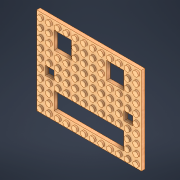
# Autodesk Inventor part: 0401_練習1
Saved by Autodesk Inventor 2022 (Build 260153000, 153)
## iProperties
Created: 2022-04-01
Part Number: 0401_練習1
Material: 一般
Document SubType Name: Modeling
Designer: User
Density: 1 g/cm^3
Appearance: 櫻桃木 - 天然低亮度
Author: User
Autodesk Inventor part; units mm, degrees
ref_plane "YZ Plane" through (0, 0, 0) normal (1, 0, 0) x (0, 1, 0)
ref_plane "XZ Plane" through (0, 0, 0) normal (0, 1, 0) x (-1, 0, 0)
ref_plane "XY Plane" through (0, 0, 0) normal (0, 0, 1) x (1, 0, 0)
sketch "草圖1" plane through (0, 0, 0) normal (0, 1, 0) x (-1, 0, 0)
  line L0 (0, 0) -> (-80, 0)
  line L1 (-80, 0) -> (-80, -96)
  line L2 (-80, -96) -> (0, -96)
  line L3 (0, -96) -> (0, 0)
  dimension "長" = 80
  dimension "寬" = 96
  constraints: 8 end point, 2 parallel, 1 horizontal, 1 perpendicular
  measures "長" distance of L2.end L1.end
  measures "寬" distance of L1.end L0.end
extrude "樂高擠出" add sketch "草圖1" against normal blind 3.2
sketch "草圖2" plane through (0, 0, 0) normal (0, 1, 0) x (-1, 0, 0)
  circle A0 centre (-76, -4) radius 2.5
  line L0 (-80, 0) -> (-80, -96) projected
  line L1 (0, 0) -> (-80, 0) projected
  dimension "d4" = 5
  dimension "d5" = 4
  dimension "d6" = 4
  constraints: 1 centre point
  measures "d4" diameter of A0
  measures "d5" distance from line of L0 A0.centre
  measures "d6" distance from line of L1 A0.centre
extrude "圓柱擠出" add sketch "草圖2" along normal blind 1.5
pattern_linear "頂部圓柱" count 12 spacing 8 along (0, 0, -1) count 10 spacing 8 along (-1, 0, 0) of "圓柱擠出"
shell "背面薄殼" thickness 1 removed faces 1 at (53.3333, -3.2, -32)
sketch "草圖3" plane through (1, -1, -1) normal (0, -1, 0) x (1, 0, 0)
  circle A0 centre (75, -3) radius 2.5 projected
  circle A1 centre (67, -3) radius 2.5 projected
  circle A2 centre (67, -11) radius 2.5 projected
  circle A3 centre (71, -7) radius 3.1569
  line L0 (78, -94) -> (0, -94) projected
  line L1 (78, -94) -> (0, -94) projected
  line L2 (78, 0) -> (78, -94) projected
  circle A4 centre (67, -19) radius 1.5 projected
  circle A5 centre (67, -11) radius 1.5 projected
  circle A6 centre (67, -3) radius 1.5 projected
  circle A7 centre (75, -19) radius 1.5 projected
  circle A8 centre (75, -11) radius 1.5 projected
  circle A9 centre (75, -3) radius 1.5 projected
  line L3 (78, 0) -> (78, -94) projected
  line L4 (0, 0) -> (78, 0) projected
  line L5 (0, -94) -> (0, 0) projected
  line L6 (78, -94) -> (0, -94) projected
  circle A10 centre (71, -15) radius 3.1569
  circle A11 centre (71, -7) radius 2.1569
  circle A12 centre (71, -15) radius 2.1569
  point P0 (-1, 1)
  dimension "d18" = 8
  dimension "d23" = 1
  dimension "d25" = 1
  constraints: 4 centre point, 3 tangent, 1 vertical, 2 other
  measures "d18" distance of A3.centre A10.centre
  measures "d23" radial gap between concentric circles of A3 A11
  measures "d25" radial gap between concentric circles of A10 A12
extrude "背面圓柱擠出" add sketch "草圖3" along normal up to surface (2.2 mm away) contours A3
pattern_linear "背面圓柱" count 11 spacing 8 along (0, 0, -1) count 9 spacing 8 along (-1, 0, 0) of "背面圓柱擠出"
sketch "草圖4" plane through (0, 0, 0) normal (0, 1, 0) x (1, 0, 0)
  circle A0 centre (8, 16) radius 2.1569 projected
  circle A1 centre (24, 32) radius 2.1569 projected
  line L0 (8, 16) -> (24, 16)
  line L1 (24, 16) -> (24, 32)
  line L2 (24, 32) -> (8, 32)
  line L3 (8, 32) -> (8, 16)
  circle A2 centre (24, 80) radius 2.1569 projected
  circle A3 centre (8, 64) radius 2.1569 projected
  line L4 (24, 80) -> (8, 80)
  line L5 (8, 80) -> (8, 64)
  line L6 (8, 64) -> (24, 64)
  line L7 (24, 64) -> (24, 80)
  circle A4 centre (72, 80) radius 2.1569 projected
  circle A5 centre (56, 16) radius 2.1569 projected
  line L8 (72, 80) -> (56, 80)
  line L9 (56, 80) -> (56, 16)
  line L10 (56, 16) -> (72, 16)
  line L11 (72, 16) -> (72, 80)
  circle A6 centre (40, 8) radius 2.1569 projected
  circle A7 centre (48, 16) radius 2.1569 projected
  line L12 (40, 8) -> (48, 8)
  line L13 (48, 8) -> (48, 16)
  line L14 (48, 16) -> (40, 16)
  line L15 (40, 16) -> (40, 8)
  circle A8 centre (40, 80) radius 2.1569 projected
  circle A9 centre (48, 88) radius 3.1569 projected
  line L16 (40, 80) -> (48, 80)
  line L17 (48, 80) -> (48, 88)
  line L18 (48, 88) -> (40, 88)
  line L19 (40, 88) -> (40, 80)
  point P0 (0, 0)
  point P1 (40, 10.1569)
  point P2 (42.1569, 8)
  point P3 (48, 13.8431)
  point P4 (45.8431, 16)
  point P5 (72, 77.8431)
  point P6 (69.8431, 80)
  point P7 (56, 18.1569)
  point P8 (58.1569, 16)
  point P9 (24, 77.8431)
  point P10 (21.8431, 80)
  point P11 (8, 66.1569)
  point P12 (10.1569, 64)
  point P13 (8, 18.1569)
  point P14 (10.1569, 16)
  point P15 (24, 29.8431)
  point P16 (21.8431, 32)
  constraints: 40 end point, 10 parallel, 5 horizontal, 5 perpendicular
extrude "表情切割" cut sketch "草圖4" along normal through all both and the other way through all contours A0 L3 L2 A1 L1 L0 | A2 L7 L6 A3 L5 L4 | A4 L11 L10 A5 L9 L8 | A6 L15 L14 A7 L13 L12 | L16 L19 A8 | A8 L19 L18 A9 L17 L16 | A9 L18 L17 picked at (40.4719, 81.3487) picked at (45.9218, 87.7658)
sketch "草圖5" plane through (1, -1, -1) normal (0, -1, 0) x (1, 0, 0)
  line L0 (47, -82.1569) -> (47, -83.8431) projected
  arc A0 (43.8431, -87) -> (47, -83.8431) centre (47, -87) ccw projected
  line L1 (43.8431, -87) -> (42.1569, -87) projected
  arc A1 (39, -83.8431) -> (42.1569, -87) centre (39, -87) ccw projected
  line L2 (39, -83.8431) -> (39, -82.1569) projected
  arc A2 (42.1569, -79) -> (39, -82.1569) centre (39, -79) ccw projected
  line L3 (42.1569, -79) -> (43.8431, -79) projected
  arc A3 (47, -82.1569) -> (43.8431, -79) centre (47, -79) ccw projected
  line L4 (43.8431, -15) -> (42.1569, -15) projected
  arc A4 (39, -11.8431) -> (42.1569, -15) centre (39, -15) ccw projected
  line L5 (39, -11.8431) -> (39, -10.1569) projected
  arc A5 (42.1569, -7) -> (39, -10.1569) centre (39, -7) ccw projected
  line L6 (42.1569, -7) -> (43.8431, -7) projected
  arc A6 (47, -10.1569) -> (43.8431, -7) centre (47, -7) ccw projected
  line L7 (47, -10.1569) -> (47, -11.8431) projected
  arc A7 (43.8431, -15) -> (47, -11.8431) centre (47, -15) ccw projected
  line L8 (11.8431, -31) -> (10.1569, -31) projected
  arc A8 (7, -27.8431) -> (10.1569, -31) centre (7, -31) ccw projected
  line L9 (7, -27.8431) -> (7, -26.1569) projected
  arc A9 (7, -19.8431) -> (7, -26.1569) centre (7, -23) ccw projected
  line L10 (7, -19.8431) -> (7, -18.1569) projected
  arc A10 (10.1569, -15) -> (7, -18.1569) centre (7, -15) ccw projected
  line L11 (10.1569, -15) -> (11.8431, -15) projected
  arc A11 (18.1569, -15) -> (11.8431, -15) centre (15, -15) ccw projected
  line L12 (18.1569, -15) -> (19.8431, -15) projected
  arc A12 (23, -18.1569) -> (19.8431, -15) centre (23, -15) ccw projected
  line L13 (23, -18.1569) -> (23, -19.8431) projected
  arc A13 (23, -26.1569) -> (23, -19.8431) centre (23, -23) ccw projected
  line L14 (23, -26.1569) -> (23, -27.8431) projected
  arc A14 (19.8431, -31) -> (23, -27.8431) centre (23, -31) ccw projected
  line L15 (19.8431, -31) -> (18.1569, -31) projected
  arc A15 (11.8431, -31) -> (18.1569, -31) centre (15, -31) ccw projected
  circle A16 centre (7, -87) radius 3.1569 projected
  circle A17 centre (7, -55) radius 3.1569 projected
  circle A18 centre (7, -47) radius 3.1569 projected
  circle A19 centre (7, -39) radius 3.1569 projected
  circle A20 centre (7, -7) radius 3.1569 projected
  circle A21 centre (15, -87) radius 3.1569 projected
  circle A22 centre (15, -55) radius 3.1569 projected
  circle A23 centre (15, -47) radius 3.1569 projected
  circle A24 centre (15, -39) radius 3.1569 projected
  circle A25 centre (15, -7) radius 3.1569 projected
  circle A26 centre (23, -87) radius 3.1569 projected
  line L16 (10.1569, -63) -> (11.8431, -63) projected
  arc A27 (18.1569, -63) -> (11.8431, -63) centre (15, -63) ccw projected
  line L17 (18.1569, -63) -> (19.8431, -63) projected
  arc A28 (23, -66.1569) -> (19.8431, -63) centre (23, -63) ccw projected
  line L18 (23, -66.1569) -> (23, -67.8431) projected
  arc A29 (23, -74.1569) -> (23, -67.8431) centre (23, -71) ccw projected
  line L19 (23, -74.1569) -> (23, -75.8431) projected
  arc A30 (19.8431, -79) -> (23, -75.8431) centre (23, -79) ccw projected
  line L20 (19.8431, -79) -> (18.1569, -79) projected
  arc A31 (11.8431, -79) -> (18.1569, -79) centre (15, -79) ccw projected
  line L21 (11.8431, -79) -> (10.1569, -79) projected
  arc A32 (7, -75.8431) -> (10.1569, -79) centre (7, -79) ccw projected
  line L22 (7, -75.8431) -> (7, -74.1569) projected
  arc A33 (7, -67.8431) -> (7, -74.1569) centre (7, -71) ccw projected
  line L23 (7, -67.8431) -> (7, -66.1569) projected
  arc A34 (10.1569, -63) -> (7, -66.1569) centre (7, -63) ccw projected
  circle A35 centre (23, -55) radius 3.1569 projected
  circle A36 centre (23, -47) radius 3.1569 projected
  circle A37 centre (23, -39) radius 3.1569 projected
  circle A38 centre (23, -7) radius 3.1569 projected
  circle A39 centre (31, -87) radius 3.1569 projected
  circle A40 centre (31, -79) radius 3.1569 projected
  circle A41 centre (31, -71) radius 3.1569 projected
  circle A42 centre (31, -63) radius 3.1569 projected
  circle A43 centre (31, -55) radius 3.1569 projected
  circle A44 centre (31, -47) radius 3.1569 projected
  circle A45 centre (31, -39) radius 3.1569 projected
  circle A46 centre (31, -31) radius 3.1569 projected
  circle A47 centre (31, -23) radius 3.1569 projected
  circle A48 centre (31, -15) radius 3.1569 projected
  circle A49 centre (31, -7) radius 3.1569 projected
  circle A50 centre (39, -71) radius 3.1569 projected
  circle A51 centre (39, -63) radius 3.1569 projected
  circle A52 centre (39, -55) radius 3.1569 projected
  circle A53 centre (39, -47) radius 3.1569 projected
  circle A54 centre (39, -39) radius 3.1569 projected
  circle A55 centre (39, -31) radius 3.1569 projected
  circle A56 centre (39, -23) radius 3.1569 projected
  circle A57 centre (47, -71) radius 3.1569 projected
  circle A58 centre (47, -63) radius 3.1569 projected
  circle A59 centre (47, -55) radius 3.1569 projected
  circle A60 centre (47, -47) radius 3.1569 projected
  circle A61 centre (47, -39) radius 3.1569 projected
  circle A62 centre (47, -31) radius 3.1569 projected
  circle A63 centre (47, -23) radius 3.1569 projected
  circle A64 centre (55, -87) radius 3.1569 projected
  circle A65 centre (55, -7) radius 3.1569 projected
  circle A66 centre (63, -87) radius 3.1569 projected
  circle A67 centre (63, -7) radius 3.1569 projected
  circle A68 centre (71, -87) radius 3.1569 projected
  line L24 (58.1569, -15) -> (59.8431, -15) projected
  arc A69 (66.1569, -15) -> (59.8431, -15) centre (63, -15) ccw projected
  line L25 (66.1569, -15) -> (67.8431, -15) projected
  arc A70 (71, -18.1569) -> (67.8431, -15) centre (71, -15) ccw projected
  line L26 (71, -18.1569) -> (71, -19.8431) projected
  arc A71 (71, -26.1569) -> (71, -19.8431) centre (71, -23) ccw projected
  line L27 (71, -26.1569) -> (71, -27.8431) projected
  arc A72 (71, -34.1569) -> (71, -27.8431) centre (71, -31) ccw projected
  line L28 (71, -34.1569) -> (71, -35.8431) projected
  arc A73 (71, -42.1569) -> (71, -35.8431) centre (71, -39) ccw projected
  line L29 (71, -42.1569) -> (71, -43.8431) projected
  arc A74 (71, -50.1569) -> (71, -43.8431) centre (71, -47) ccw projected
  line L30 (71, -50.1569) -> (71, -51.8431) projected
  arc A75 (71, -58.1569) -> (71, -51.8431) centre (71, -55) ccw projected
  line L31 (71, -58.1569) -> (71, -59.8431) projected
  arc A76 (71, -66.1569) -> (71, -59.8431) centre (71, -63) ccw projected
  line L32 (71, -66.1569) -> (71, -67.8431) projected
  arc A77 (71, -74.1569) -> (71, -67.8431) centre (71, -71) ccw projected
  line L33 (71, -74.1569) -> (71, -75.8431) projected
  arc A78 (67.8431, -79) -> (71, -75.8431) centre (71, -79) ccw projected
  line L34 (67.8431, -79) -> (66.1569, -79) projected
  arc A79 (59.8431, -79) -> (66.1569, -79) centre (63, -79) ccw projected
  line L35 (59.8431, -79) -> (58.1569, -79) projected
  arc A80 (55, -75.8431) -> (58.1569, -79) centre (55, -79) ccw projected
  line L36 (55, -75.8431) -> (55, -74.1569) projected
  arc A81 (55, -67.8431) -> (55, -74.1569) centre (55, -71) ccw projected
  line L37 (55, -67.8431) -> (55, -66.1569) projected
  arc A82 (55, -59.8431) -> (55, -66.1569) centre (55, -63) ccw projected
  line L38 (55, -59.8431) -> (55, -58.1569) projected
  arc A83 (55, -51.8431) -> (55, -58.1569) centre (55, -55) ccw projected
  line L39 (55, -51.8431) -> (55, -50.1569) projected
  arc A84 (55, -43.8431) -> (55, -50.1569) centre (55, -47) ccw projected
  line L40 (55, -43.8431) -> (55, -42.1569) projected
  arc A85 (55, -35.8431) -> (55, -42.1569) centre (55, -39) ccw projected
  line L41 (55, -35.8431) -> (55, -34.1569) projected
  arc A86 (55, -27.8431) -> (55, -34.1569) centre (55, -31) ccw projected
  line L42 (55, -27.8431) -> (55, -26.1569) projected
  arc A87 (55, -19.8431) -> (55, -26.1569) centre (55, -23) ccw projected
  line L43 (55, -19.8431) -> (55, -18.1569) projected
  arc A88 (58.1569, -15) -> (55, -18.1569) centre (55, -15) ccw projected
  line L44 (78, 0) -> (78, -94) projected
  line L45 (0, 0) -> (78, 0) projected
  line L46 (0, -94) -> (0, 0) projected
  line L47 (78, -94) -> (0, -94) projected
  circle A89 centre (75, -3) radius 1.5 projected
  circle A90 centre (75, -11) radius 1.5 projected
  circle A91 centre (75, -19) radius 1.5 projected
  circle A92 centre (75, -27) radius 1.5 projected
  circle A93 centre (75, -35) radius 1.5 projected
  circle A94 centre (75, -43) radius 1.5 projected
  circle A95 centre (75, -51) radius 1.5 projected
  circle A96 centre (75, -59) radius 1.5 projected
  circle A97 centre (75, -67) radius 1.5 projected
  circle A98 centre (75, -75) radius 1.5 projected
  circle A99 centre (75, -83) radius 1.5 projected
  circle A100 centre (75, -91) radius 1.5 projected
  circle A101 centre (67, -3) radius 1.5 projected
  circle A102 centre (67, -11) radius 1.5 projected
  circle A103 centre (67, -83) radius 1.5 projected
  circle A104 centre (67, -91) radius 1.5 projected
  circle A105 centre (59, -3) radius 1.5 projected
  circle A106 centre (59, -11) radius 1.5 projected
  circle A107 centre (59, -83) radius 1.5 projected
  circle A108 centre (59, -91) radius 1.5 projected
  circle A109 centre (51, -3) radius 1.5 projected
  circle A110 centre (51, -11) radius 1.5 projected
  circle A111 centre (51, -19) radius 1.5 projected
  circle A112 centre (51, -27) radius 1.5 projected
  circle A113 centre (51, -35) radius 1.5 projected
  circle A114 centre (51, -43) radius 1.5 projected
  circle A115 centre (51, -51) radius 1.5 projected
  circle A116 centre (51, -59) radius 1.5 projected
  circle A117 centre (51, -67) radius 1.5 projected
  circle A118 centre (51, -75) radius 1.5 projected
  circle A119 centre (51, -83) radius 1.5 projected
  circle A120 centre (51, -91) radius 1.5 projected
  circle A121 centre (43, -3) radius 1.5 projected
  circle A122 centre (43, -19) radius 1.5 projected
  circle A123 centre (43, -27) radius 1.5 projected
  circle A124 centre (43, -35) radius 1.5 projected
  circle A125 centre (43, -43) radius 1.5 projected
  circle A126 centre (43, -51) radius 1.5 projected
  circle A127 centre (43, -59) radius 1.5 projected
  circle A128 centre (43, -67) radius 1.5 projected
  circle A129 centre (43, -75) radius 1.5 projected
  circle A130 centre (43, -91) radius 1.5 projected
  circle A131 centre (35, -3) radius 1.5 projected
  circle A132 centre (35, -11) radius 1.5 projected
  circle A133 centre (35, -19) radius 1.5 projected
  circle A134 centre (35, -27) radius 1.5 projected
  circle A135 centre (35, -35) radius 1.5 projected
  circle A136 centre (35, -43) radius 1.5 projected
  circle A137 centre (35, -51) radius 1.5 projected
  circle A138 centre (35, -59) radius 1.5 projected
  circle A139 centre (35, -67) radius 1.5 projected
  circle A140 centre (35, -75) radius 1.5 projected
  circle A141 centre (35, -83) radius 1.5 projected
  circle A142 centre (35, -91) radius 1.5 projected
  circle A143 centre (27, -3) radius 1.5 projected
  circle A144 centre (27, -11) radius 1.5 projected
  circle A145 centre (27, -19) radius 1.5 projected
  circle A146 centre (27, -27) radius 1.5 projected
  circle A147 centre (27, -35) radius 1.5 projected
  circle A148 centre (27, -43) radius 1.5 projected
  circle A149 centre (27, -51) radius 1.5 projected
  circle A150 centre (27, -59) radius 1.5 projected
  circle A151 centre (27, -67) radius 1.5 projected
  circle A152 centre (27, -75) radius 1.5 projected
  circle A153 centre (27, -83) radius 1.5 projected
  circle A154 centre (27, -91) radius 1.5 projected
  circle A155 centre (19, -3) radius 1.5 projected
  circle A156 centre (19, -11) radius 1.5 projected
  circle A157 centre (19, -35) radius 1.5 projected
  circle A158 centre (19, -43) radius 1.5 projected
  circle A159 centre (19, -51) radius 1.5 projected
  circle A160 centre (19, -59) radius 1.5 projected
  circle A161 centre (19, -83) radius 1.5 projected
  circle A162 centre (19, -91) radius 1.5 projected
  circle A163 centre (11, -3) radius 1.5 projected
  circle A164 centre (11, -11) radius 1.5 projected
  circle A165 centre (11, -35) radius 1.5 projected
  circle A166 centre (11, -43) radius 1.5 projected
  circle A167 centre (11, -51) radius 1.5 projected
  circle A168 centre (11, -59) radius 1.5 projected
  circle A169 centre (11, -83) radius 1.5 projected
  circle A170 centre (11, -91) radius 1.5 projected
  circle A171 centre (3, -3) radius 1.5 projected
  circle A172 centre (3, -11) radius 1.5 projected
  circle A173 centre (3, -19) radius 1.5 projected
  circle A174 centre (3, -27) radius 1.5 projected
  circle A175 centre (3, -35) radius 1.5 projected
  circle A176 centre (3, -43) radius 1.5 projected
  circle A177 centre (3, -51) radius 1.5 projected
  circle A178 centre (3, -59) radius 1.5 projected
  circle A179 centre (3, -67) radius 1.5 projected
  circle A180 centre (3, -75) radius 1.5 projected
  circle A181 centre (3, -83) radius 1.5 projected
  circle A182 centre (3, -91) radius 1.5 projected
  circle A183 centre (71, -7) radius 3.1569 projected
  line L48 (23, -79) -> (7, -79)
  line L49 (7, -79) -> (7, -63)
  line L50 (7, -63) -> (23, -63)
  line L51 (23, -63) -> (23, -79)
  line L52 (27, -83) -> (3, -83)
  line L53 (3, -83) -> (3, -59)
  line L54 (3, -59) -> (27, -59)
  line L55 (27, -59) -> (27, -83)
  line L56 (39, -81.1569) -> (39, -79) projected
  line L57 (47, -84.8431) -> (47, -87) projected
  line L58 (39, -79) -> (47, -79)
  line L59 (47, -79) -> (47, -87)
  line L60 (47, -87) -> (39, -87)
  line L61 (39, -87) -> (39, -79)
  circle A184 centre (35, -91) radius 1.5 projected
  circle A185 centre (51, -75) radius 1.5 projected
  line L62 (35, -91) -> (51, -91)
  line L63 (51, -91) -> (51, -75)
  line L64 (51, -75) -> (35, -75)
  line L65 (35, -75) -> (35, -91)
  line L66 (71, -79) -> (55, -79)
  line L67 (55, -79) -> (55, -15)
  line L68 (55, -15) -> (71, -15)
  line L69 (71, -15) -> (71, -79)
  line L70 (75, -11) -> (51, -11)
  line L71 (51, -11) -> (51, -83)
  line L72 (51, -83) -> (75, -83)
  line L73 (75, -83) -> (75, -11)
  arc A186 (44.8431, -15) -> (47, -12.8431) centre (47, -15) ccw projected
  line L74 (47, -15) -> (39, -15)
  line L75 (39, -15) -> (39, -7)
  line L76 (39, -7) -> (47, -7)
  line L77 (47, -7) -> (47, -15)
  line L78 (51, -19) -> (35, -19)
  line L79 (35, -19) -> (35, -3)
  line L80 (35, -3) -> (51, -3)
  line L81 (51, -3) -> (51, -19)
  arc A187 (9.1569, -15) -> (7, -17.1569) centre (7, -15) ccw projected
  line L82 (23, -31) -> (7, -31)
  line L83 (7, -31) -> (7, -15)
  line L84 (7, -15) -> (23, -15)
  line L85 (23, -15) -> (23, -31)
  circle A188 centre (27, -11) radius 1.5 projected
  circle A189 centre (3, -35) radius 1.5 projected
  line L86 (27, -11) -> (3, -11)
  line L87 (3, -11) -> (3, -35)
  line L88 (3, -35) -> (27, -35)
  line L89 (27, -35) -> (27, -11)
  arc A190 (23, -76.8431) -> (20.8431, -79) centre (23, -79) ccw projected
  arc A191 (7, -65.1569) -> (9.1569, -63) centre (7, -63) ccw projected
  arc A192 (71, -76.8431) -> (68.8431, -79) centre (71, -79) ccw projected
  arc A193 (55, -17.1569) -> (57.1569, -15) centre (55, -15) ccw projected
  arc A194 (39, -9.1569) -> (41.1569, -7) centre (39, -7) ccw projected
  arc A195 (47, -12.8431) -> (44.8431, -15) centre (47, -15) ccw projected
  arc A196 (7, -17.1569) -> (9.1569, -15) centre (7, -15) ccw projected
  arc A197 (23, -28.8431) -> (20.8431, -31) centre (23, -31) ccw projected
  point P0 (-1, 1)
  point P1 (35, -84.5)
  point P2 (35, -89.5)
  point P3 (36.5, -91)
  point P4 (41.5, -91)
  point P5 (44.5, -91)
  point P6 (49.5, -91)
  point P7 (51, -89.5)
  point P8 (51, -84.5)
  point P9 (52.5, -83)
  point P10 (57.5, -83)
  point P11 (60.5, -83)
  point P12 (65.5, -83)
  point P13 (68.5, -83)
  point P14 (73.5, -83)
  point P15 (75, -81.5)
  point P16 (75, -76.5)
  point P17 (75, -73.5)
  point P18 (75, -68.5)
  point P19 (75, -65.5)
  point P20 (75, -60.5)
  point P21 (75, -57.5)
  point P22 (75, -52.5)
  point P23 (75, -49.5)
  point P24 (75, -44.5)
  point P25 (75, -41.5)
  point P26 (75, -36.5)
  point P27 (75, -33.5)
  point P28 (75, -28.5)
  point P29 (75, -25.5)
  point P30 (75, -20.5)
  point P31 (75, -17.5)
  point P32 (75, -12.5)
  point P33 (73.5, -11)
  point P34 (68.5, -11)
  point P35 (65.5, -11)
  point P36 (60.5, -11)
  point P37 (57.5, -11)
  point P38 (52.5, -11)
  point P39 (51, -12.5)
  point P40 (51, -17.5)
  point P41 (51, -20.5)
  point P42 (51, -25.5)
  point P43 (51, -28.5)
  point P44 (51, -33.5)
  point P45 (51, -36.5)
  point P46 (51, -41.5)
  point P47 (51, -44.5)
  point P48 (51, -49.5)
  point P49 (51, -52.5)
  point P50 (51, -57.5)
  point P51 (51, -60.5)
  point P52 (51, -65.5)
  point P53 (51, -68.5)
  point P54 (51, -73.5)
  point P55 (49.5, -75)
  point P56 (44.5, -75)
  point P57 (41.5, -75)
  point P58 (36.5, -75)
  point P59 (35, -76.5)
  point P60 (35, -81.5)
  point P61 (27, -81.5)
  point P62 (27, -76.5)
  point P63 (27, -73.5)
  point P64 (27, -68.5)
  point P65 (27, -65.5)
  point P66 (27, -60.5)
  point P67 (25.5, -59)
  point P68 (20.5, -59)
  point P69 (17.5, -59)
  point P70 (12.5, -59)
  point P71 (9.5, -59)
  point P72 (4.5, -59)
  point P73 (3, -60.5)
  point P74 (3, -65.5)
  point P75 (3, -68.5)
  point P76 (3, -73.5)
  point P77 (3, -76.5)
  point P78 (3, -81.5)
  point P79 (4.5, -83)
  point P80 (9.5, -83)
  point P81 (12.5, -83)
  point P82 (17.5, -83)
  point P83 (20.5, -83)
  point P84 (25.5, -83)
  point P85 (27, -33.5)
  point P86 (27, -28.5)
  point P87 (27, -25.5)
  point P88 (27, -20.5)
  point P89 (27, -17.5)
  point P90 (27, -12.5)
  point P91 (25.5, -11)
  point P92 (20.5, -11)
  point P93 (17.5, -11)
  point P94 (12.5, -11)
  point P95 (9.5, -11)
  point P96 (4.5, -11)
  point P97 (3, -12.5)
  point P98 (3, -17.5)
  point P99 (3, -20.5)
  point P100 (3, -25.5)
  point P101 (3, -28.5)
  point P102 (3, -33.5)
  point P103 (4.5, -35)
  point P104 (9.5, -35)
  point P105 (12.5, -35)
  point P106 (17.5, -35)
  point P107 (20.5, -35)
  point P108 (25.5, -35)
  point P109 (10.1569, -15)
  point P110 (18.1569, -15)
  point P111 (51, -9.5)
  point P112 (51, -4.5)
  point P113 (49.5, -3)
  point P114 (44.5, -3)
  point P115 (41.5, -3)
  point P116 (36.5, -3)
  point P117 (35, -4.5)
  point P118 (35, -9.5)
  point P119 (35, -12.5)
  point P120 (35, -17.5)
  point P121 (36.5, -19)
  point P122 (41.5, -19)
  point P123 (44.5, -19)
  point P124 (49.5, -19)
  point P125 (18.1569, -63)
  constraints: 80 end point, 20 parallel, 10 horizontal, 10 perpendicular, 1 coincident, 1 midpoint
extrude "表情切割修補" cut sketch "草圖5" along normal mid plane 10 contours A195 L77 L74 | L75 L76 A194 | A197 L85 L82 | L83 L84 A196 | A191 L49 L50 | L51 L48 A190 | A193 L67 L68 | L69 L66 A192
extrude "背面修齊" add sketch "草圖5" along normal up to surface (2.2 mm away) contours L59 L58 A3 | A0 L60 L57 L59 | L58 L56 L61 A2 | A1 L61 L60 | L74 A186 L77 A7 | A4 L75 L74 | L74 L77 A186 | L77 L76 A6 | A5 L76 L75 | L82 A15 | A8 L83 L82 | L82 L85 A14 | A9 L83 | L85 A13 | A10 L84 A187 L83 | A187 L84 L83 | L85 L84 A12 | A11 L84 | L50 L49 A34 | A27 L50 | L49 A33 | A28 L51 L50 | L49 L48 A32 | A29 L51 | L48 A31 | A30 L48 L51 | L68 L67 A88 | A69 L68 | L67 A87 | A70 L69 L68 | L67 A86 | A71 L69 | L67 A85 | A72 L69 | L67 A84 | A73 L69 | L67 A83 | A74 L69 | L67 A82 | A75 L69 | L67 A81 | A76 L69 | L67 L66 A80 | A77 L69 | L66 A79 | A78 L66 L69 | A90 L73 A91 A92 A93 A94 A95 A96 A97 A98 A99 L72 A103 A107 A119 L63 A118 L71 A117 A116 A115 A114 A113 A112 A111 A110 L70 A106 A102 | A110 L71 A111 L78 A122 A133 L79 A132 A131 L80 A121 A109 L81 | A118 L63 A119 A120 L62 A130 A142 L65 A141 A140 L64 A129 | A144 L89 A145 A146 A147 L88 A157 A165 A175 L87 A174 A173 A172 L86 A164 A156 | A150 L55 A151 A152 A153 L52 A161 A169 A181 L53 A180 A179 A178 L54 A168 A160
